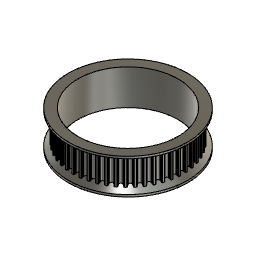
TimingPulleyBase (Autodesk Fusion 360 design; units mm, degrees)
Autodesk Fusion 360 part; units mm, degrees
sketch "Sketch1" plane through (0, 0, 0) normal (0, 0, 1) x (1, 0, 0)
  circle A0 centre (0, 0) radius 15.6615
  circle A1 centre (0, 0) radius 14.1615
  dimension "dd1" = 31.323
  constraint coincident A0.centre A1.centre
  measures "dd1" diameter of A0
extrude "Extrude1" add sketch "Sketch1" along normal blind 10
sketch "Sketch2" plane through (0, 0, 10) normal (0, 0, 1) x (-1, 0, 0)
  circle A0 centre (0, 0) radius 14.1615
  circle A1 centre (0, 0) radius 15.6615
  circle A2 centre (0, 0) radius 15.9155 construction
  circle A3 centre (0, 0) radius 15.6615
  line L0 (0, 0) -> (-8.5944, 0) construction
  arc A4 (-15.2982, 0.54) -> (-15.5149, 0.5963) centre (-15.6565, -0.3936) ccw
  line L1 (-15.4665, 0) -> (-15.1403, 0.449) construction
  line L2 (-15.6565, -0.3936) -> (-15.2982, 0.54) construction
  arc A5 (-14.9115, 0) -> (-15.1403, 0.449) centre (-15.4665, 0) ccw
  arc A6 (-15.6434, 0.752) -> (-15.5149, 0.5963) centre (-15.4936, 0.7448) ccw
  line L3 (0, 0) -> (-15.6565, -0.3936) construction
  line L4 (-15.1403, 0.449) -> (-9.7436, -3.4719) construction
  line L5 (-15.2982, 0.54) -> (-8.7886, -1.9588) construction
  spline S0 degree 5 poles (-15.1403, 0.449) (-15.1421, 0.4503) (-15.1479, 0.4542) (-15.1635, 0.4638) (-15.1952, 0.4826) (-15.2415, 0.5095) (-15.2736, 0.5276) (-15.2898, 0.5362) (-15.2961, 0.5392) (-15.2982, 0.54) knots 0 0 0 0 0 0 0.2 0.4 0.6 0.8 1 1 1 1 1 1
  line L6 (-15.1364, 0.4462) -> (-15.1442, 0.4519)
  line L7 (-15.2937, 0.5382) -> (-15.3027, 0.5417)
  arc A7 (-15.1403, -0.449) -> (-14.9115, 0) centre (-15.4665, 0) ccw
  spline S1 degree 5 poles (-15.1403, -0.449) (-15.1421, -0.4503) (-15.1479, -0.4542) (-15.1635, -0.4638) (-15.1952, -0.4826) (-15.2415, -0.5095) (-15.2736, -0.5276) (-15.2898, -0.5362) (-15.2961, -0.5392) (-15.2982, -0.54) knots 0 0 0 0 0 0 0.2 0.4 0.6 0.8 1 1 1 1 1 1
  line L8 (-15.1364, -0.4462) -> (-15.1442, -0.4519)
  line L9 (-15.2937, -0.5382) -> (-15.3027, -0.5417)
  arc A8 (-15.5149, -0.5963) -> (-15.2982, -0.54) centre (-15.6565, 0.3936) ccw
  arc A9 (-15.5149, -0.5963) -> (-15.6434, -0.752) centre (-15.4936, -0.7448) ccw
  line L10 (-15.4665, 0) -> (-15.1442, 0.4519) construction
  point P0 (-14.9115, 0)
  point P1 (-15.4665, 0)
  dimension "d187" = 31.831
  dimension "d191" = 31.323
  dimension "d192" = 14.9115
  dimension "d196" = 0.555
  dimension "d198" = 1
  dimension "d202" = 54
  dimension "d203" = 69
  dimension "d204" = 0.555
  dimension "d205" = 0.15
  dimension "d208" = 1.44
  dimension "d211" = 54.5
  constraint coincident A0.centre A1.centre
  constraint horizontal L0
  constraint coincident L0 P0
  constraint coincident L0 P1
  constraint coincident P1 L1.start
  constraint coincident A4.centre L2.start
  constraint coincident P0 A5.start
  constraint coincident L1.end A5.end
  constraint tangent A4 A6
  constraint coincident A3 A4.centre
  constraint coincident A4.start L2.end
  constraint tangent A3 A6
  constraint coincident A3 A6.start
  constraint tangent A4 L5
  constraint tangent A5 L4
  constraint midpoint L1.end L6
  constraint parallel L4 L6
  constraint midpoint A4.start L7
  constraint symmetric L0 A4.end A8.start
  constraint symmetric L0 A4 A8
  constraint symmetric L0 A4.start S1.end
  constraint symmetric L0 L1.end A7.start
  constraint symmetric L0 P0 A5.start
  constraint symmetric L0 A5 A7
  constraint symmetric L0 A6.start A9.end
  constraint symmetric L0 A6 A9
  constraint symmetric L0 L6.start L8.start
  constraint symmetric L0 L6.end L8.end
  constraint symmetric L0 L7.start L9.start
  constraint symmetric L0 L7.end L9.end
  constraint equal L6 L7
  constraint coincident L6.end L10.end
  constraint parallel L5 L7
  measures "d187" diameter of A2
  measures "d191" diameter of A3
  measures "d192" distance of A0.centre P0
  measures "d196" distance of P0 P1
  measures "d198" radius of A4
  measures "d202" angle of L0 L1
  measures "d203" angle of L0 L2
  measures "d204" radius of A5
  measures "d205" radius of A6
  measures "d208" angle of L0 L3
  measures "d211" angle of L0 L10
extrude "Extrude2" cut sketch "Sketch2" along normal mid plane 24 contours A1 A3 A4 A5 A6 S0 L6 L7 A7 S1 L8 L9 A8 A9 picked at (-15.4102, 0)
pattern_circular "C-Pattern1" count 50 over 360 about axis through (0, 0, 1.75) along (0, 0, 1) of "Extrude2"
sketch "Sketch5" plane through (0, 0, 0) normal (0, 1, 0) x (1, 0, 0)
  line L0 (0, -0.6) -> (14.1615, -0.6) construction
  line L1 (14.1615, -0.6) -> (14.9115, -0.6) construction
  line L2 (14.9115, -0.6) -> (14.9115, -2) construction
  line L3 (14.9115, -2) -> (14.9115, -8) construction
  line L4 (14.9115, -8) -> (14.9115, -9.4) construction
  line L5 (14.1615, -0.6) -> (14.1615, -9.4)
  line L6 (14.1615, -0.6) -> (14.9115, -0.6) construction
  line L7 (14.9115, -9.4) -> (16.9109, -9.4) construction
  line L8 (14.9115, -0.6) -> (16.9109, -0.6)
  line L9 (16.9109, -9.4) -> (14.9115, -8)
  line L10 (16.9109, -0.6) -> (14.9115, -2)
  line L11 (14.9115, -2) -> (14.1615, -2)
  line L12 (14.9115, -8) -> (14.1615, -8)
  line L13 (14.9115, -9.4) -> (14.1615, -9.4) construction
  line L14 (0, 0) -> (0, -0.6) construction
  line L15 (14.1615, -0.6) -> (16.9109, -0.6)
  line L16 (16.9109, -0.6) -> (16.9109, 0)
  line L17 (16.9109, 0) -> (14.1615, 0)
  line L18 (14.1615, 0) -> (14.1615, -0.6)
  line L19 (14.1615, -9.4) -> (16.9109, -9.4)
  line L20 (16.9109, -9.4) -> (16.9109, -10)
  line L21 (16.9109, -10) -> (14.1615, -10)
  line L22 (14.1615, -10) -> (14.1615, -9.4)
  line L23 (0, -0.6) -> (15.6615, -0.6) construction
  dimension "d58" = 14.1615
  dimension "d60" = 1.4
  dimension "d61" = 6
  dimension "d62" = 1.4
  dimension "d64" = 0.75
  dimension "d68" = 0.6
  dimension "d69" = 0.6
  dimension "d70" = 0.6
  dimension "d71" = 55
  dimension "d72" = 55
  dimension "d73" = 15.6615
  constraint horizontal L0
  constraint parallel L0 L1
  constraint perpendicular L1 L2
  constraint parallel L2 L3
  constraint parallel L3 L4
  constraint perpendicular L0 L5
  constraint perpendicular L4 L7
  constraint perpendicular L2 L8
  constraint coincident L5 L11.end
  constraint perpendicular L5 L11
  constraint coincident L5 L12.end
  constraint perpendicular L5 L12
  constraint collinear L7 L13
  constraint coincident L14.start origin
  constraint perpendicular L0 L14
  constraint horizontal L15
  constraint vertical L16
  constraint horizontal L17
  constraint vertical L18
  constraint horizontal L19
  constraint vertical L20
  constraint horizontal L21
  constraint vertical L22
  constraint perpendicular L14 L23
  measures "d58" distance of L0.start L0.end
  measures "d60" distance of L1.end L2.end
  measures "d61" distance of L2.end L3.end
  measures "d62" distance of L3.end L4.end
  measures "d64" distance of L0.end L1.end
  measures "d68" distance of L0.start L14.start
  measures "d69" distance of L0.end L17.end
  measures "d70" distance of L5.end L21.end
  measures "d71" angle of L3 L9
  measures "d72" angle of L3 L10
  measures "d73" distance of L0.start L23.end
revolve "Revolve1" add sketch "Sketch5" angle 360 about axis through (0, 0, 1.75) along (0, 0, 1)
equation "nTeeth = 50" comment "Number of teeth on the large pulley"
equation "p = 2 mm" comment "Belt parameter pitch"
equation "r1 = 0.15 mm" comment "Belt parameter R1"
equation "r2 = 1.00 mm" comment "Belt parameter R2"
equation "r3 = 0.555 mm" comment "Belt parameter R3"
equation "b = 0.40 mm" comment "Belt parameter b"
equation "hTotal = 1.38 mm" comment "Belt parameter total Height"
equation "h = 0.75 mm" comment "Belt parameter tooth height h"
equation "i = 0.63 mm" comment "Belt parameter back thickness"
equation "pld = 0.254 mm" comment "Belt parameter pld"
equation "dd1 = largeDiameter - 2 * pld"
equation "d22 = -pulleyThickness"
equation "d23 = beltWidth + 2 * beltPadding"
equation "beltWidth = 6 mm"
equation "beltPadding = 2 mm"
equation "pulleyThickness = 1.5 mm" comment "Thickness for pulley, should be greater than h"
equation "d42 = 2 * beltWidth"
equation "d44 = nTeeth"
equation "d58 = dd1 / 2 - pulleyThickness"
equation "d60 = beltPadding - minSpacing * 2"
equation "d61 = beltWidth"
equation "d62 = beltPadding - minSpacing * 2"
equation "d64 = pulleyThickness - h"
equation "minSpacing = 0.3 mm"
equation "d68 = minSpacing * 2"
equation "d69 = minSpacing * 2"
equation "d70 = minSpacing * 2"
equation "d71 = ledgeAngle"
equation "d72 = d71"
equation "d73 = ( dd1 / 2 )"
equation "largeDiameter = p * nTeeth / PI"
equation "ledgeAngle = 55 deg" comment "overhang angle for ledge"
equation "d187 = largeDiameter"
equation "d191 = largeDiameter - ( 2 * pld )"
equation "d192 = largeDiameter / 2 - ( pld + h )"
equation "d196 = r3"
equation "d198 = r2"
equation "d204 = r3"
equation "d205 = r1"
equation "d208 = asin(b / ( largeDiameter / 2 ))"
equation "d211 = d202 + 0.5 deg"
